Autodesk Inventor part; units mm, degrees
(part 3 of 6)
sketch "S06_305p5" plane through (0, 0, 0) normal (0, 0, 1) x (1, 0, 0)
  spline S0 degree 4 poles (213.0067, -18.9729) (212.9621, -18.9593) (212.7441, -18.8914) (212.3779, -18.779) (211.76, -18.589) (211.1099, -18.3887) (210.3111, -18.1449) (209.3704, -17.8569) (208.2858, -17.5275) (207.06, -17.1556) (205.6934, -16.744) (204.1871, -16.2917) (202.5432, -15.8012) (200.7622, -15.273) (198.8468, -14.7079) (196.7975, -14.1085) (194.6171, -13.4749) (192.3074, -12.8093) (189.8703, -12.1119) (187.3078, -11.3857) (184.6228, -10.6315) (181.8175, -9.8511) (178.8941, -9.0457) (175.8563, -8.2172) (172.7057, -7.3673) (169.4465, -6.4982) (166.0803, -5.6102) (162.6118, -4.7065) (159.0427, -3.7875) (155.3779, -2.8566) (151.6194, -1.9137) (147.7719, -0.9621) (143.8383, -0.0025) (139.823, 0.9626) (135.7291, 1.9321) (131.5615, 2.9039) (127.3228, 3.876) (123.0184, 4.8472) (118.6519, 5.8151) (114.2273, 6.7786) (109.7493, 7.7354) (105.2217, 8.684) (100.6494, 9.6229) (96.037, 10.5501) (91.388, 11.4635) (86.7084, 12.362) (82.0012, 13.2442) (77.2724, 14.1069) (72.5256, 14.9504) (67.7665, 15.7715) (62.9985, 16.5699) (58.2276, 17.3431) (53.4575, 18.0889) (48.6936, 18.8084) (43.9401, 19.497) (39.198, 20.1563) (34.4798, 20.7818) (29.764, 21.3777) (25.0643, 21.9267) (20.3983, 22.4316) (15.7673, 22.8898) (11.1792, 23.3003) (6.6388, 23.6643) (2.1513, 23.9785) (-2.2794, 24.2462) (-6.6474, 24.4635) (-10.9492, 24.6332) (-15.1794, 24.7536) (-19.3341, 24.8266) (-23.4084, 24.8507) (-27.3984, 24.828) (-31.2994, 24.7581) (-35.1072, 24.6427) (-38.8184, 24.4813) (-42.4284, 24.2766) (-45.9333, 24.0285) (-49.3303, 23.7389) (-52.6149, 23.4083) (-55.7842, 23.0395) (-58.8346, 22.6326) (-61.7632, 22.1892) (-64.5669, 21.7125) (-67.2427, 21.2022) (-69.788, 20.6607) (-72.2009, 20.0906) (-74.4779, 19.492) (-76.6177, 18.8678) (-78.6179, 18.2193) (-80.477, 17.548) (-82.1928, 16.8552) (-83.7647, 16.1431) (-85.1908, 15.4128) (-86.47, 14.6646) (-87.6028, 13.9015) (-88.5865, 13.1217) (-89.4223, 12.3271) (-90.1087, 11.5175) (-90.6444, 10.6919) (-91.026, 9.8504) (-91.2528, 8.9963) (-91.3206, 8.1309) (-91.2339, 7.2672) (-90.9897, 6.4183) (-90.5915, 5.5855) (-90.0424, 4.771) (-89.3451, 3.9743) (-88.5017, 3.1953) (-87.5133, 2.4322) (-86.3813, 1.6851) (-85.1065, 0.9538) (-83.6901, 0.2383) (-82.1338, -0.4608) (-80.4387, -1.1438) (-78.6069, -1.8099) (-76.64, -2.4594) (-74.5405, -3.091) (-72.3099, -3.7061) (-69.951, -4.3022) (-67.4659, -4.8811) (-64.8574, -5.442) (-62.1277, -5.9843) (-59.28, -6.5077) (-56.3167, -7.0143) (-53.2411, -7.5009) (-50.0561, -7.9709) (-46.7643, -8.422) (-43.3697, -8.8561) (-39.875, -9.2733) (-36.2838, -9.6725) (-32.5993, -10.0572) (-28.825, -10.4242) (-24.9649, -10.7779) (-21.0222, -11.1159) (-17.0003, -11.4409) (-12.9041, -11.7535) (-8.7359, -12.0531) (-4.5012, -12.3424) (-0.2027, -12.6213) (4.1549, -12.8906) (8.5679, -13.1521) (13.0318, -13.4068) (17.5428, -13.6542) (22.0992, -13.8979) (26.6939, -14.135) (31.334, -14.3737) (36.0271, -14.6) (40.7407, -14.8159) (45.4804, -15.0198) (50.2352, -15.2139) (55.002, -15.3986) (59.7756, -15.5745) (64.5509, -15.7416) (69.3235, -15.9018) (74.0888, -16.0537) (78.842, -16.2004) (83.5783, -16.3396) (88.2931, -16.4744) (92.9816, -16.6035) (97.6397, -16.727) (102.2619, -16.8472) (106.8441, -16.9625) (111.3818, -17.0733) (115.8706, -17.1813) (120.3053, -17.2848) (124.6826, -17.3854) (128.9972, -17.4825) (133.245, -17.576) (137.4219, -17.6663) (141.5241, -17.7536) (145.5464, -17.838) (149.4858, -17.9187) (153.338, -17.9962) (157.0988, -18.0714) (160.7646, -18.1421) (164.332, -18.2107) (167.7969, -18.2752) (171.156, -18.3377) (174.406, -18.3956) (177.5435, -18.4513) (180.565, -18.5032) (183.468, -18.5523) (186.2488, -18.5977) (188.9052, -18.641) (191.434, -18.6801) (193.8328, -18.7171) (196.0991, -18.7511) (198.2305, -18.7816) (200.2247, -18.81) (202.08, -18.836) (203.7939, -18.8588) (205.3647, -18.8797) (206.7912, -18.8976) (208.0711, -18.9142) (209.2039, -18.9279) (210.1875, -18.9398) (211.0222, -18.9501) (211.7026, -18.9575) (212.349, -18.9658) (212.7318, -18.9695) (212.96, -18.9722) (213.0067, -18.9729) knots 0 0 0 0 0 0.003306 0.005253 0.00752 0.010062 0.01285 0.015861 0.019079 0.022488 0.026078 0.029837 0.033757 0.037828 0.042045 0.046398 0.050884 0.055494 0.060224 0.065069 0.070023 0.075082 0.080241 0.085495 0.090841 0.096274 0.101791 0.107386 0.113057 0.118799 0.124609 0.130484 0.136419 0.142412 0.148458 0.154554 0.160697 0.166884 0.17311 0.179374 0.185671 0.191998 0.198352 0.20473 0.211128 0.217543 0.223972 0.230412 0.23686 0.243312 0.249765 0.256217 0.262663 0.2691 0.275526 0.281941 0.288345 0.294734 0.301105 0.307451 0.313767 0.320049 0.326294 0.332498 0.338659 0.344773 0.350837 0.356848 0.362801 0.368695 0.374525 0.380288 0.38598 0.391599 0.39714 0.4026 0.407976 0.413263 0.418458 0.423557 0.428556 0.433452 0.438241 0.442917 0.447478 0.451919 0.456236 0.460425 0.464482 0.468403 0.472185 0.475825 0.479322 0.482675 0.485889 0.48897 0.49193 0.494788 0.497572 0.50031 0.503032 0.505769 0.508552 0.511409 0.514365 0.517441 0.520647 0.523991 0.527474 0.531098 0.534861 0.538758 0.542789 0.546947 0.551231 0.555634 0.560154 0.564786 0.569527 0.574371 0.579315 0.584356 0.58949 0.594712 0.60002 0.605409 0.610877 0.61642 0.622034 0.627716 0.633463 0.639271 0.645138 0.651061 0.657035 0.663059 0.669128 0.675241 0.681393 0.687582 0.693804 0.700057 0.706341 0.712655 0.718998 0.725365 0.731751 0.738149 0.744556 0.750969 0.757385 0.7638 0.770211 0.776616 0.783011 0.789393 0.795759 0.802106 0.808429 0.814727 0.820996 0.827232 0.833433 0.839595 0.845714 0.851788 0.857813 0.863785 0.869702 0.875558 0.881352 0.887078 0.892735 0.898316 0.90382 0.909242 0.914577 0.919822 0.924972 0.930023 0.93497 0.939808 0.944533 0.949139 0.95362 0.95797 0.962183 0.966252 0.970169 0.973927 0.977515 0.980924 0.984141 0.987151 0.989939 0.99248 0.994747 0.996694 1 1 1 1 1
  circle A0 centre (0, 0) radius 5.15
  line L0 (-70.9, 8.1) -> (-60.7, 8.1)
  line L1 (-60.7, 8.1) -> (-60.7, 3.9)
  line L2 (-60.7, 3.9) -> (-70.9, 3.9)
  line L3 (-70.9, 3.9) -> (-70.9, 8.1)
  line L4 (-70.9, 8.1) -> (-60.7, 3.9) construction
  line L5 (-60.7, 8.1) -> (-70.9, 3.9) construction
  line L6 (-35.65, 7.1) -> (-25.45, 7.1)
  line L7 (-25.45, 7.1) -> (-25.45, 2.9)
  line L8 (-25.45, 2.9) -> (-35.65, 2.9)
  line L9 (-35.65, 2.9) -> (-35.65, 7.1)
  line L10 (-35.65, 7.1) -> (-25.45, 2.9) construction
  line L11 (-25.45, 7.1) -> (-35.65, 2.9) construction
  line L12 (120.1, -1.9) -> (109.9, -1.9)
  line L13 (109.9, -1.9) -> (109.9, -6.1)
  line L14 (109.9, -6.1) -> (120.1, -6.1)
  line L15 (120.1, -6.1) -> (120.1, -1.9)
  line L16 (120.1, -1.9) -> (109.9, -6.1) construction
  line L17 (109.9, -1.9) -> (120.1, -6.1) construction
  line L18 (59.1, -4.6) -> (48.9, -4.6)
  line L19 (48.9, -4.6) -> (48.9, -0.4)
  line L20 (48.9, -0.4) -> (59.1, -0.4)
  line L21 (59.1, -0.4) -> (59.1, -4.6)
  line L22 (59.1, -4.6) -> (48.9, -0.4) construction
  line L23 (48.9, -4.6) -> (59.1, -0.4) construction
  point P0 (212.7151, -18.8828)
  point P1 (212.3506, -18.7706)
  point P2 (211.841, -18.6139)
  point P3 (211.1866, -18.4126)
  point P4 (210.3879, -18.1682)
  point P5 (209.4456, -17.8803)
  point P6 (208.3604, -17.5502)
  point P7 (207.1336, -17.1784)
  point P8 (205.7662, -16.7662)
  point P9 (204.2591, -16.3139)
  point P10 (202.6141, -15.8229)
  point P11 (200.8323, -15.2943)
  point P12 (198.9157, -14.7292)
  point P13 (196.8654, -14.1291)
  point P14 (194.6838, -13.4953)
  point P15 (192.3729, -12.8291)
  point P16 (189.9344, -12.1316)
  point P17 (187.3706, -11.4048)
  point P18 (184.6842, -10.6503)
  point P19 (181.8775, -9.8693)
  point P20 (178.9527, -9.0635)
  point P21 (175.9131, -8.2345)
  point P22 (172.761, -7.3842)
  point P23 (169.5, -6.5144)
  point P24 (166.1323, -5.6262)
  point P25 (162.6618, -4.7217)
  point P26 (159.091, -3.8025)
  point P27 (155.4242, -2.8708)
  point P28 (151.6639, -1.9276)
  point P29 (147.8143, -0.9753)
  point P30 (143.8788, -0.0153)
  point P31 (139.8614, 0.9504)
  point P32 (135.7655, 1.9204)
  point P33 (131.5956, 2.8927)
  point P34 (127.3548, 3.8654)
  point P35 (123.0481, 4.837)
  point P36 (118.6794, 5.8055)
  point P37 (114.2526, 6.7693)
  point P38 (109.7722, 7.7266)
  point P39 (105.2423, 8.6757)
  point P40 (100.6677, 9.615)
  point P41 (96.0527, 10.5426)
  point P42 (91.4016, 11.4565)
  point P43 (86.7194, 12.3554)
  point P44 (82.0099, 13.2377)
  point P45 (77.2786, 14.1011)
  point P46 (72.5295, 14.9446)
  point P47 (67.7677, 15.7663)
  point P48 (62.9974, 16.5647)
  point P49 (58.2239, 17.338)
  point P50 (53.4515, 18.0845)
  point P51 (48.6851, 18.8035)
  point P52 (43.9294, 19.4928)
  point P53 (39.1892, 20.1511)
  point P54 (34.4692, 20.777)
  point P55 (29.7515, 21.3699)
  point P56 (25.0468, 21.9203)
  point P57 (20.3755, 22.425)
  point P58 (15.742, 22.8831)
  point P59 (11.1516, 23.2938)
  point P60 (6.6091, 23.657)
  point P61 (2.1192, 23.9717)
  point P62 (-2.3135, 24.2383)
  point P63 (-6.6837, 24.4558)
  point P64 (-10.9875, 24.6247)
  point P65 (-15.2198, 24.745)
  point P66 (-19.3763, 24.8171)
  point P67 (-23.4525, 24.841)
  point P68 (-27.4443, 24.8174)
  point P69 (-31.347, 24.747)
  point P70 (-35.1566, 24.6306)
  point P71 (-38.8693, 24.4687)
  point P72 (-42.4807, 24.2628)
  point P73 (-45.9871, 24.0139)
  point P74 (-49.3853, 23.7231)
  point P75 (-52.6712, 23.3916)
  point P76 (-55.8415, 23.0213)
  point P77 (-58.8928, 22.6131)
  point P78 (-61.8222, 22.1686)
  point P79 (-64.6265, 21.6899)
  point P80 (-67.3027, 21.1781)
  point P81 (-69.8483, 20.635)
  point P82 (-72.2609, 20.0626)
  point P83 (-74.5378, 19.4621)
  point P84 (-76.6767, 18.8356)
  point P85 (-78.6759, 18.1846)
  point P86 (-80.5332, 17.5106)
  point P87 (-82.2468, 16.8151)
  point P88 (-83.8155, 16.1001)
  point P89 (-85.2374, 15.3667)
  point P90 (-86.5115, 14.6162)
  point P91 (-87.6369, 13.8503)
  point P92 (-88.6122, 13.0695)
  point P93 (-89.4371, 12.2753)
  point P94 (-90.111, 11.4689)
  point P95 (-90.6333, 10.6504)
  point P96 (-91.0034, 9.821)
  point P97 (-91.2221, 8.981)
  point P98 (-91.2886, 8.1312)
  point P99 (-91.2037, 7.283)
  point P100 (-90.9677, 6.448)
  point P101 (-90.5814, 5.6265)
  point P102 (-90.0455, 4.8188)
  point P103 (-89.3605, 4.025)
  point P104 (-88.5275, 3.246)
  point P105 (-87.5476, 2.4815)
  point P106 (-86.4222, 1.732)
  point P107 (-85.1524, 0.9978)
  point P108 (-83.7399, 0.2794)
  point P109 (-82.1864, -0.4227)
  point P110 (-80.4934, -1.1084)
  point P111 (-78.663, -1.7772)
  point P112 (-76.6971, -2.4289)
  point P113 (-74.5981, -3.0631)
  point P114 (-72.3677, -3.6798)
  point P115 (-70.0087, -4.2782)
  point P116 (-67.5233, -4.8587)
  point P117 (-64.9143, -5.4212)
  point P118 (-62.1839, -5.9649)
  point P119 (-59.3353, -6.4901)
  point P120 (-56.3711, -6.9973)
  point P121 (-53.2944, -7.4858)
  point P122 (-50.1082, -7.9564)
  point P123 (-46.8152, -8.4089)
  point P124 (-43.4191, -8.8439)
  point P125 (-39.9231, -9.2617)
  point P126 (-36.3304, -9.6624)
  point P127 (-32.6443, -10.0471)
  point P128 (-28.8684, -10.4156)
  point P129 (-25.0065, -10.7694)
  point P130 (-21.0621, -11.1085)
  point P131 (-17.0385, -11.4341)
  point P132 (-12.9402, -11.747)
  point P133 (-8.7703, -12.0476)
  point P134 (-4.5334, -12.3372)
  point P135 (-0.2331, -12.6166)
  point P136 (4.1267, -12.8865)
  point P137 (8.5417, -13.1485)
  point P138 (13.0077, -13.4034)
  point P139 (17.5206, -13.6517)
  point P140 (22.0763, -13.8949)
  point P141 (26.6704, -14.1336)
  point P142 (31.3138, -14.3696)
  point P143 (36.0095, -14.5968)
  point P144 (40.7302, -14.8127)
  point P145 (45.4721, -15.0173)
  point P146 (50.2296, -15.2116)
  point P147 (54.9987, -15.3966)
  point P148 (59.7748, -15.5726)
  point P149 (64.5525, -15.7402)
  point P150 (69.3275, -15.9003)
  point P151 (74.0952, -16.0529)
  point P152 (78.8509, -16.1992)
  point P153 (83.5897, -16.3391)
  point P154 (88.3068, -16.4737)
  point P155 (92.9978, -16.603)
  point P156 (97.6582, -16.727)
  point P157 (102.2829, -16.8469)
  point P158 (106.8674, -16.9624)
  point P159 (111.4075, -17.0736)
  point P160 (115.8986, -17.1813)
  point P161 (120.3357, -17.2852)
  point P162 (124.7151, -17.3857)
  point P163 (129.032, -17.4828)
  point P164 (133.282, -17.5765)
  point P165 (137.4612, -17.6668)
  point P166 (141.5654, -17.7542)
  point P167 (145.5899, -17.8385)
  point P168 (149.5313, -17.9193)
  point P169 (153.3856, -17.997)
  point P170 (157.1484, -18.0718)
  point P171 (160.8161, -18.143)
  point P172 (164.3853, -18.2113)
  point P173 (167.8521, -18.2762)
  point P174 (171.213, -18.3382)
  point P175 (174.4648, -18.3966)
  point P176 (177.6039, -18.452)
  point P177 (180.6271, -18.5041)
  point P178 (183.5316, -18.553)
  point P179 (186.314, -18.5987)
  point P180 (188.9718, -18.6416)
  point P181 (191.502, -18.6811)
  point P182 (193.9021, -18.7179)
  point P183 (196.1696, -18.7518)
  point P184 (198.3022, -18.7826)
  point P185 (200.2976, -18.811)
  point P186 (202.1539, -18.8368)
  point P187 (203.8689, -18.8598)
  point P188 (205.4407, -18.8805)
  point P189 (206.8681, -18.8987)
  point P190 (208.149, -18.915)
  point P191 (209.2826, -18.9288)
  point P192 (210.2676, -18.9408)
  point P193 (211.1025, -18.9508)
  point P194 (211.7873, -18.9587)
  point P195 (212.3204, -18.9651)
  point P196 (212.7015, -18.9693)
  point P197 (212.9304, -18.9719)
  point P198 (-65.8, 6)
  point P199 (-30.55, 5)
  dimension "d10" = 10.3
  dimension "d11" = 91.65
  dimension "d69" = 10.2
  dimension "d70" = 4.2
  dimension "d72" = 10.2
  dimension "d73" = 4.2
  dimension "d142" = 65.8
  dimension "d143" = 6
  dimension "d144" = 0
  dimension "d145" = 30.55
  dimension "d146" = 5
  dimension "d227" = 10.2
  dimension "d228" = 4.2
  dimension "d229" = 115
  dimension "d230" = 4
  dimension "d231" = 10.2
  dimension "d232" = 4.2
  dimension "d233" = 54
  dimension "d234" = 2.5
  constraints: 48 end point, 8 midpoint, 8 parallel, 4 horizontal, 4 perpendicular, 1 centre point, 201 other
  measures "d10" diameter of A0
  measures "d11" distance of A0.centre point (-91.289, 8.131)
  measures "d69" distance of L1.end L2.end
  measures "d70" distance of L0.end L1.end
  measures "d72" distance of L7.end L8.end
  measures "d73" distance of L6.end L7.end
  measures "d142" horizontal distance of point (0, 0) point (-65.8, 6)
  measures "d143" vertical distance of A0.centre point (-65.8, 6)
  measures "d144" distance of point (0, 0) A0.centre
  measures "d145" horizontal distance of point (0, 0) point (-30.55, 5)
  measures "d146" vertical distance of point (0, 0) point (-30.55, 5)
  measures "d227" distance of L14.end L13.end
  measures "d228" distance of L13.end L12.end
  measures "d229" horizontal distance of point (0, 0) point (115, -4)
  measures "d230" vertical distance of point (115, -4) point (0, 0)
  measures "d231" distance of L19.end L20.end
  measures "d232" distance of L18.end L19.end
  measures "d233" horizontal distance of point (54, -2.5) point (0, 0)
  measures "d234" vertical distance of point (0, 0) point (54, -2.5)
sketch "S07_285p6" plane through (0, 0, 0) normal (0, 0, 1) x (1, 0, 0)
  spline S0 degree 4 poles (198.678, -22.2502) (198.6365, -22.2366) (198.4342, -22.1685) (198.0944, -22.0557) (197.5209, -21.865) (196.9176, -21.664) (196.1762, -21.4192) (195.3031, -21.13) (194.2964, -20.7992) (193.1586, -20.4256) (191.8901, -20.0119) (190.4919, -19.5573) (188.9658, -19.0639) (187.3125, -18.5325) (185.5343, -17.9638) (183.6317, -17.3601) (181.6073, -16.7216) (179.4627, -16.0506) (177.1997, -15.3471) (174.8202, -14.614) (172.3267, -13.8522) (169.7214, -13.0633) (167.0062, -12.2486) (164.1846, -11.4098) (161.258, -10.5486) (158.2303, -9.6672) (155.103, -8.7659) (151.8805, -7.8477) (148.5642, -6.9131) (145.1587, -5.9654) (141.666, -5.0044) (138.0902, -4.0334) (134.4342, -3.0531) (130.7019, -2.0659) (126.8961, -1.073) (123.0216, -0.0763) (119.0807, 0.9221) (115.0783, 1.9211) (111.0178, 2.9184) (106.9029, 3.9127) (102.738, 4.9019) (98.5265, 5.8845) (94.2731, 6.859) (89.9818, 7.8235) (85.6562, 8.7757) (81.3016, 9.7147) (76.9209, 10.6391) (72.5196, 11.5457) (68.101, 12.4347) (63.6704, 13.3031) (59.2311, 14.1504) (54.7886, 14.9742) (50.3461, 15.7725) (45.9089, 16.5459) (41.4808, 17.2904) (37.0628, 18.0071) (32.6663, 18.6918) (28.2715, 19.3488) (23.8906, 19.9616) (19.5404, 20.5324) (15.2219, 21.0589) (10.9425, 21.5399) (6.7067, 21.9763) (2.5193, 22.3652) (-1.6161, 22.7093) (-5.6939, 23.0051) (-9.7109, 23.2549) (-13.662, 23.4572) (-17.5435, 23.6135) (-21.3509, 23.7225) (-25.0805, 23.7859) (-28.7279, 23.8033) (-32.2893, 23.7762) (-35.7612, 23.7041) (-39.1395, 23.5893) (-42.4206, 23.4317) (-45.6016, 23.2331) (-48.6785, 22.9938) (-51.6484, 22.7163) (-54.508, 22.4008) (-57.2545, 22.0485) (-59.885, 21.6624) (-62.3967, 21.2422) (-64.7871, 20.7901) (-67.0543, 20.3084) (-69.1952, 19.7973) (-71.2083, 19.2592) (-73.0915, 18.6956) (-74.8433, 18.1076) (-76.4615, 17.4965) (-77.9458, 16.8643) (-79.2942, 16.212) (-80.5056, 15.5398) (-81.5805, 14.8506) (-82.5165, 14.1427) (-83.3144, 13.4177) (-83.9732, 12.6757) (-84.4913, 11.9154) (-84.8658, 11.137) (-85.0959, 10.3436) (-85.1776, 9.5362) (-85.1149, 8.7271) (-84.9046, 7.9286) (-84.5502, 7.1417) (-84.0543, 6.3688) (-83.4195, 5.6094) (-82.6477, 4.8635) (-81.7401, 4.1293) (-80.698, 3.407) (-79.522, 2.6965) (-78.2134, 1.9977) (-76.7737, 1.3113) (-75.2039, 0.637) (-73.506, -0.0244) (-71.6815, -0.6731) (-69.7326, -1.308) (-67.6609, -1.9301) (-65.4689, -2.5373) (-63.1585, -3.1311) (-60.7325, -3.7106) (-58.1927, -4.2754) (-55.5423, -4.8249) (-52.7835, -5.3613) (-49.9193, -5.8813) (-46.9525, -6.3881) (-43.8855, -6.8795) (-40.722, -7.3572) (-37.4646, -7.8213) (-34.1167, -8.2706) (-30.6813, -8.7082) (-27.1615, -9.1313) (-23.5613, -9.5438) (-19.8835, -9.9433) (-16.1315, -10.3323) (-12.3098, -10.7113) (-8.4204, -11.0798) (-4.4687, -11.44) (-0.4572, -11.7918) (3.6099, -12.1359) (7.7288, -12.4739) (11.8955, -12.8067) (16.1063, -13.1336) (20.3596, -13.4579) (24.6488, -13.7771) (28.9806, -14.0985) (33.362, -14.4096) (37.7628, -14.7113) (42.1883, -15.0025) (46.6281, -15.2847) (51.0794, -15.5584) (55.5372, -15.8241) (59.9967, -16.0815) (64.4539, -16.3324) (68.9044, -16.5755) (73.3437, -16.8134) (77.7674, -17.044) (82.1711, -17.2699) (86.5503, -17.4901) (90.9013, -17.7043) (95.2187, -17.9147) (99.4989, -18.1196) (103.7376, -18.3194) (107.9306, -18.5156) (112.0732, -18.7063) (116.1622, -18.8932) (120.1926, -19.0755) (124.1607, -19.253) (128.0626, -19.4259) (131.8948, -19.5946) (135.6523, -19.7587) (139.3324, -19.9177) (142.9311, -20.0718) (146.4444, -20.2218) (149.869, -20.3657) (153.2017, -20.5055) (156.4387, -20.6393) (159.5769, -20.7689) (162.6132, -20.8919) (165.5444, -21.0105) (168.3673, -21.1232) (171.0794, -21.2306) (173.6774, -21.332) (176.1593, -21.4289) (178.5219, -21.519) (180.7631, -21.6044) (182.8805, -21.6844) (184.8719, -21.758) (186.7351, -21.8269) (188.4685, -21.8905) (190.0699, -21.9481) (191.5376, -22.0011) (192.8705, -22.0481) (194.0663, -22.0907) (195.1248, -22.1275) (196.0438, -22.1595) (196.8237, -22.1868) (197.4594, -22.2081) (198.0634, -22.2296) (198.4212, -22.2412) (198.6343, -22.2486) (198.678, -22.2502) knots 0 0 0 0 0 0.003306 0.005253 0.00752 0.010062 0.01285 0.015861 0.019079 0.022488 0.026078 0.029837 0.033757 0.037828 0.042045 0.046398 0.050884 0.055494 0.060224 0.065069 0.070023 0.075082 0.080241 0.085495 0.090841 0.096274 0.101791 0.107386 0.113057 0.118799 0.124609 0.130484 0.136419 0.142412 0.148458 0.154554 0.160697 0.166884 0.17311 0.179374 0.185671 0.191998 0.198352 0.20473 0.211128 0.217543 0.223972 0.230412 0.23686 0.243312 0.249765 0.256217 0.262663 0.2691 0.275526 0.281941 0.288345 0.294734 0.301105 0.307451 0.313767 0.320049 0.326294 0.332498 0.338659 0.344773 0.350837 0.356848 0.362801 0.368695 0.374525 0.380288 0.38598 0.391599 0.39714 0.4026 0.407976 0.413263 0.418458 0.423557 0.428556 0.433452 0.438241 0.442917 0.447478 0.451919 0.456236 0.460425 0.464482 0.468403 0.472185 0.475825 0.479322 0.482675 0.485889 0.48897 0.49193 0.494788 0.497572 0.50031 0.503032 0.505769 0.508552 0.511409 0.514365 0.517441 0.520647 0.523991 0.527474 0.531098 0.534861 0.538758 0.542789 0.546947 0.551231 0.555634 0.560154 0.564786 0.569527 0.574371 0.579315 0.584356 0.58949 0.594712 0.60002 0.605409 0.610877 0.61642 0.622034 0.627716 0.633463 0.639271 0.645138 0.651061 0.657035 0.663059 0.669128 0.675241 0.681393 0.687582 0.693804 0.700057 0.706341 0.712655 0.718998 0.725365 0.731751 0.738149 0.744556 0.750969 0.757385 0.7638 0.770211 0.776616 0.783011 0.789393 0.795759 0.802106 0.808429 0.814727 0.820996 0.827232 0.833433 0.839595 0.845714 0.851788 0.857813 0.863785 0.869702 0.875558 0.881352 0.887078 0.892735 0.898316 0.90382 0.909242 0.914577 0.919822 0.924972 0.930023 0.93497 0.939808 0.944533 0.949139 0.95362 0.95797 0.962183 0.966252 0.970169 0.973927 0.977515 0.980924 0.984141 0.987151 0.989939 0.99248 0.994747 0.996694 1 1 1 1 1
  circle A0 centre (0, 0) radius 5.15
  line L0 (-25.45, 2.9) -> (-35.65, 2.9)
  line L1 (-35.65, 2.9) -> (-35.65, 7.1)
  line L2 (-35.65, 7.1) -> (-25.45, 7.1)
  line L3 (-25.45, 7.1) -> (-25.45, 2.9)
  line L4 (-25.45, 2.9) -> (-35.65, 7.1) construction
  line L5 (-35.65, 2.9) -> (-25.45, 7.1) construction
  line L6 (-62.22, 12.1) -> (-52.02, 12.1)
  line L7 (-52.02, 12.1) -> (-52.02, 7.9)
  line L8 (-52.02, 7.9) -> (-62.22, 7.9)
  line L9 (-62.22, 7.9) -> (-62.22, 12.1)
  line L10 (-62.22, 12.1) -> (-52.02, 7.9) construction
  line L11 (-52.02, 12.1) -> (-62.22, 7.9) construction
  line L12 (48.9, -0.4) -> (59.1, -0.4)
  line L13 (59.1, -0.4) -> (59.1, -4.6)
  line L14 (59.1, -4.6) -> (48.9, -4.6)
  line L15 (48.9, -4.6) -> (48.9, -0.4)
  line L16 (48.9, -0.4) -> (59.1, -4.6) construction
  line L17 (59.1, -0.4) -> (48.9, -4.6) construction
  line L18 (105.1, -12.1) -> (94.9, -12.1)
  line L19 (94.9, -12.1) -> (94.9, -7.9)
  line L20 (94.9, -7.9) -> (105.1, -7.9)
  line L21 (105.1, -7.9) -> (105.1, -12.1)
  line L22 (105.1, -12.1) -> (94.9, -7.9) construction
  line L23 (94.9, -12.1) -> (105.1, -7.9) construction
  point P0 (198.4073, -22.1598)
  point P1 (198.069, -22.0472)
  point P2 (197.5961, -21.8899)
  point P3 (196.9887, -21.688)
  point P4 (196.2475, -21.4426)
  point P5 (195.3729, -21.1535)
  point P6 (194.3656, -20.822)
  point P7 (193.2269, -20.4485)
  point P8 (191.9576, -20.0342)
  point P9 (190.5587, -19.5795)
  point P10 (189.0316, -19.0858)
  point P11 (187.3775, -18.5539)
  point P12 (185.5982, -17.9851)
  point P13 (183.6947, -17.3808)
  point P14 (181.6692, -16.7421)
  point P15 (179.5235, -16.0705)
  point P16 (177.2592, -15.3668)
  point P17 (174.8785, -14.6332)
  point P18 (172.3837, -13.871)
  point P19 (169.777, -13.0816)
  point P20 (167.0606, -12.2664)
  point P21 (164.2373, -11.4272)
  point P22 (161.3093, -10.5656)
  point P23 (158.2799, -9.6835)
  point P24 (155.1513, -8.7819)
  point P25 (151.9268, -7.863)
  point P26 (148.6091, -6.9281)
  point P27 (145.2017, -5.9795)
  point P28 (141.7073, -5.0183)
  point P29 (138.1295, -4.0466)
  point P30 (134.4717, -3.0659)
  point P31 (130.7374, -2.0781)
  point P32 (126.9299, -1.0847)
  point P33 (123.0532, -0.0875)
  point P34 (119.1104, 0.9115)
  point P35 (115.1058, 1.9109)
  point P36 (111.0433, 2.9088)
  point P37 (106.9264, 3.9035)
  point P38 (102.7592, 4.8932)
  point P39 (98.5456, 5.8764)
  point P40 (94.29, 6.8513)
  point P41 (89.9964, 7.8161)
  point P42 (85.6688, 8.7689)
  point P43 (81.3118, 9.7083)
  point P44 (76.9289, 10.6328)
  point P45 (72.5252, 11.5402)
  point P46 (68.1045, 12.4292)
  point P47 (63.6714, 13.2981)
  point P48 (59.23, 14.1456)
  point P49 (54.785, 14.9696)
  point P50 (50.3404, 15.7685)
  point P51 (45.9009, 16.5416)
  point P52 (41.4707, 17.2866)
  point P53 (37.0544, 18.0025)
  point P54 (32.6563, 18.6876)
  point P55 (28.2596, 19.3418)
  point P56 (23.8741, 19.9559)
  point P57 (19.5189, 20.5267)
  point P58 (15.1981, 21.0531)
  point P59 (10.9165, 21.5343)
  point P60 (6.6787, 21.9701)
  point P61 (2.4891, 22.3595)
  point P62 (-1.6482, 22.7027)
  point P63 (-5.7281, 22.9986)
  point P64 (-9.7468, 23.2478)
  point P65 (-13.6999, 23.45)
  point P66 (-17.5831, 23.6055)
  point P67 (-21.3923, 23.7143)
  point P68 (-25.1236, 23.777)
  point P69 (-28.7727, 23.7939)
  point P70 (-32.3357, 23.7659)
  point P71 (-35.8091, 23.6933)
  point P72 (-39.1888, 23.5775)
  point P73 (-42.4712, 23.4192)
  point P74 (-45.6534, 23.2195)
  point P75 (-48.7314, 22.9794)
  point P76 (-51.7023, 22.7005)
  point P77 (-54.5628, 22.3838)
  point P78 (-57.3101, 22.0304)
  point P79 (-59.9412, 21.6426)
  point P80 (-62.4533, 21.2209)
  point P81 (-64.844, 20.7673)
  point P82 (-67.111, 20.2835)
  point P83 (-69.2517, 19.7706)
  point P84 (-71.2641, 19.2304)
  point P85 (-73.1464, 18.6644)
  point P86 (-74.8966, 18.0738)
  point P87 (-76.5129, 17.4602)
  point P88 (-77.9942, 16.8251)
  point P89 (-79.3387, 16.1699)
  point P90 (-80.5454, 15.4955)
  point P91 (-81.6135, 14.8035)
  point P92 (-82.5416, 14.0944)
  point P93 (-83.3294, 13.3696)
  point P94 (-83.9764, 12.6302)
  point P95 (-84.4818, 11.8764)
  point P96 (-84.8454, 11.109)
  point P97 (-85.0675, 10.3286)
  point P98 (-85.1477, 9.5358)
  point P99 (-85.0864, 8.7412)
  point P100 (-84.8835, 7.9558)
  point P101 (-84.5399, 7.1799)
  point P102 (-84.0561, 6.4135)
  point P103 (-83.4327, 5.6572)
  point P104 (-82.6707, 4.9114)
  point P105 (-81.7711, 4.1761)
  point P106 (-80.7352, 3.4517)
  point P107 (-79.564, 2.7386)
  point P108 (-78.2591, 2.0372)
  point P109 (-76.8221, 1.3481)
  point P110 (-75.2543, 0.6713)
  point P111 (-73.5578, 0.0074)
  point P112 (-71.7342, -0.6434)
  point P113 (-69.7858, -1.2806)
  point P114 (-67.7144, -1.9043)
  point P115 (-65.5223, -2.5136)
  point P116 (-63.2117, -3.1089)
  point P117 (-60.7852, -3.6899)
  point P118 (-58.2448, -4.2561)
  point P119 (-55.5937, -4.8073)
  point P120 (-52.834, -5.3443)
  point P121 (-49.9688, -5.866)
  point P122 (-47.0009, -6.3734)
  point P123 (-43.9328, -6.8662)
  point P124 (-40.768, -7.3447)
  point P125 (-37.5093, -7.8094)
  point P126 (-34.16, -8.2601)
  point P127 (-30.7231, -8.6979)
  point P128 (-27.2019, -9.1224)
  point P129 (-23.6, -9.535)
  point P130 (-19.9206, -9.9355)
  point P131 (-16.167, -10.3251)
  point P132 (-12.3433, -10.7045)
  point P133 (-8.4524, -11.0739)
  point P134 (-4.4987, -11.4345)
  point P135 (-0.4854, -11.7868)
  point P136 (3.5835, -12.1315)
  point P137 (7.7044, -12.47)
  point P138 (11.873, -12.803)
  point P139 (16.0856, -13.1307)
  point P140 (20.3382, -13.4547)
  point P141 (24.6269, -13.7752)
  point P142 (28.9617, -14.0943)
  point P143 (33.3456, -14.4062)
  point P144 (37.7531, -14.7081)
  point P145 (42.1806, -14.9999)
  point P146 (46.623, -15.2824)
  point P147 (51.0764, -15.5564)
  point P148 (55.5364, -15.8223)
  point P149 (59.9982, -16.0803)
  point P150 (64.4577, -16.3311)
  point P151 (68.9104, -16.5749)
  point P152 (73.3521, -16.8125)
  point P153 (77.7781, -17.0438)
  point P154 (82.184, -17.2696)
  point P155 (86.5655, -17.4899)
  point P156 (90.9186, -17.7047)
  point P157 (95.2383, -17.9149)
  point P158 (99.5207, -18.12)
  point P159 (103.7616, -18.3202)
  point P160 (107.9567, -18.5161)
  point P161 (112.1016, -18.7073)
  point P162 (116.1925, -18.8942)
  point P163 (120.2251, -19.0765)
  point P164 (124.1953, -19.2542)
  point P165 (128.0993, -19.4273)
  point P166 (131.9334, -19.596)
  point P167 (135.693, -19.7601)
  point P168 (139.3749, -19.9193)
  point P169 (142.9755, -20.0736)
  point P170 (146.4907, -20.2233)
  point P171 (149.9172, -20.3676)
  point P172 (153.2516, -20.5071)
  point P173 (156.4903, -20.6414)
  point P174 (159.6302, -20.7706)
  point P175 (162.6681, -20.8941)
  point P176 (165.6009, -21.0125)
  point P177 (168.4253, -21.1253)
  point P178 (171.1388, -21.2326)
  point P179 (173.7383, -21.3344)
  point P180 (176.2215, -21.4308)
  point P181 (178.5854, -21.5214)
  point P182 (180.8278, -21.6067)
  point P183 (182.9464, -21.6865)
  point P184 (184.9389, -21.7605)
  point P185 (186.8032, -21.8293)
  point P186 (188.5377, -21.8928)
  point P187 (190.14, -21.9507)
  point P188 (191.6086, -22.0034)
  point P189 (192.9423, -22.0507)
  point P190 (194.1391, -22.0931)
  point P191 (195.1983, -22.1301)
  point P192 (196.1186, -22.1622)
  point P193 (196.8987, -22.1892)
  point P194 (197.5386, -22.2111)
  point P195 (198.0367, -22.2284)
  point P196 (198.3928, -22.2404)
  point P197 (198.6067, -22.2477)
  point P198 (-30.55, 5)
  point P199 (-57.12, 10)
  dimension "d12" = 10.3
  dimension "d13" = 85.68
  dimension "d75" = 10.2
  dimension "d76" = 4.2
  dimension "d78" = 10.2
  dimension "d79" = 4.2
  dimension "d147" = 30.55
  dimension "d148" = 5
  dimension "d149" = 57.12
  dimension "d150" = 10
  dimension "d235" = 10.2
  dimension "d236" = 4.2
  dimension "d237" = 54
  dimension "d238" = 2.5
  dimension "d239" = 10.2
  dimension "d240" = 4.2
  dimension "d241" = 100
  dimension "d242" = 10
  constraints: 48 end point, 8 midpoint, 8 parallel, 4 horizontal, 4 perpendicular, 1 centre point, 201 other
  measures "d12" diameter of A0
  measures "d13" distance of A0.centre point (-85.148, 9.536)
  measures "d75" distance of L1.end L2.end
  measures "d76" distance of L0.end L1.end
  measures "d78" distance of L7.end L8.end
  measures "d79" distance of L6.end L7.end
  measures "d147" horizontal distance of point (0, 0) point (-30.55, 5)
  measures "d148" vertical distance of point (0, 0) point (-30.55, 5)
  measures "d149" horizontal distance of point (0, 0) point (-57.12, 10)
  measures "d150" vertical distance of point (0, 0) point (-57.12, 10)
  measures "d235" distance of L13.end L14.end
  measures "d236" distance of L12.end L13.end
  measures "d237" horizontal distance of point (0, 0) point (54, -2.5)
  measures "d238" vertical distance of point (0, 0) point (54, -2.5)
  measures "d239" distance of L19.end L20.end
  measures "d240" distance of L18.end L19.end
  measures "d241" horizontal distance of point (100, -10) point (0, 0)
  measures "d242" vertical distance of point (0, 0) point (100, -10)
sketch "S08_271p4" plane through (0, 0, 0) normal (0, 0, 1) x (1, 0, 0)
  spline S0 degree 4 poles (187.5255, -30.4397) (187.4869, -30.4248) (187.298, -30.3507) (186.9808, -30.2277) (186.4454, -30.0198) (185.8822, -29.8007) (185.19, -29.5336) (184.375, -29.2182) (183.435, -28.857) (182.3726, -28.449) (181.188, -27.9968) (179.8823, -27.4997) (178.457, -26.9599) (176.9127, -26.3779) (175.2517, -25.7547) (173.4742, -25.0924) (171.5828, -24.3915) (169.5788, -23.6539) (167.4639, -22.8801) (165.2399, -22.0727) (162.909, -21.2326) (160.4732, -20.3617) (157.9345, -19.461) (155.2958, -18.5325) (152.5584, -17.5778) (149.7261, -16.5992) (146.8003, -15.597) (143.7848, -14.5743) (140.6811, -13.5317) (137.4934, -12.4724) (134.2234, -11.3964) (130.8751, -10.3071) (127.4511, -9.2051) (123.955, -8.0931) (120.3895, -6.9721) (116.7589, -5.8443) (113.0653, -4.7118) (109.3133, -3.5759) (105.5063, -2.4388) (101.6474, -1.302) (97.7408, -0.1678) (93.7897, 0.9625) (89.7984, 2.0869) (85.7707, 3.2037) (81.7099, 4.3104) (77.6209, 5.4059) (73.5064, 6.4889) (69.3716, 7.5558) (65.2195, 8.6069) (61.0551, 9.639) (56.8814, 10.6514) (52.7036, 11.6418) (48.5246, 12.6079) (44.3494, 13.5501) (40.1815, 14.4645) (36.0219, 15.352) (31.8812, 16.2082) (27.7409, 17.0379) (23.6116, 17.825) (19.5095, 18.5709) (15.4354, 19.2732) (11.3964, 19.9305) (7.3966, 20.5435) (3.4404, 21.1091) (-0.4684, 21.6297) (-4.3249, 22.1017) (-8.1257, 22.5274) (-11.8663, 22.9047) (-15.543, 23.2352) (-19.1515, 23.5172) (-22.6884, 23.7524) (-26.1495, 23.9401) (-29.5309, 24.0814) (-32.8296, 24.1759) (-36.0414, 24.2254) (-39.1629, 24.2298) (-42.1914, 24.1906) (-45.1229, 24.1078) (-47.9548, 23.9838) (-50.6837, 23.8184) (-53.307, 23.6129) (-55.8218, 23.3699) (-58.2254, 23.0889) (-60.5154, 22.772) (-62.6898, 22.4212) (-64.7458, 22.0365) (-66.6817, 21.6203) (-68.4955, 21.1737) (-70.1858, 20.6978) (-71.7504, 20.1937) (-73.1888, 19.6633) (-74.4991, 19.1075) (-75.6805, 18.5264) (-76.733, 17.9227) (-77.6546, 17.2946) (-78.446, 16.644) (-79.106, 15.9706) (-79.6335, 15.2733) (-80.0254, 14.5521) (-80.281, 13.8098) (-80.3965, 13.0474) (-80.3749, 12.2765) (-80.2128, 11.5087) (-79.9133, 10.7452) (-79.4789, 9.9884) (-78.912, 9.2379) (-78.2145, 8.4937) (-77.3875, 7.7543) (-76.4323, 7.0199) (-75.3495, 6.2903) (-74.1403, 5.5657) (-72.806, 4.8467) (-71.3477, 4.133) (-69.7673, 3.4256) (-68.066, 2.7243) (-66.2461, 2.0303) (-64.3089, 1.3426) (-62.257, 0.6634) (-60.092, -0.0085) (-57.8166, -0.6724) (-55.4325, -1.3276) (-52.9428, -1.9735) (-50.3495, -2.612) (-47.6554, -3.2399) (-44.8633, -3.8601) (-41.9754, -4.4705) (-38.9953, -5.0723) (-35.9254, -5.6656) (-32.7689, -6.2491) (-29.5288, -6.8257) (-26.208, -7.3924) (-22.8103, -7.9527) (-19.3384, -8.5045) (-15.7955, -9.0497) (-12.186, -9.5888) (-8.5118, -10.121) (-4.778, -10.6483) (-0.9872, -11.1704) (2.8568, -11.6878) (6.7503, -12.2019) (10.6894, -12.7132) (14.6706, -13.221) (18.6923, -13.7284) (22.7483, -14.2326) (26.8446, -14.7409) (30.9885, -15.2417) (35.1513, -15.7345) (39.338, -16.2185) (43.5386, -16.6947) (47.7506, -17.1633) (51.9691, -17.6246) (56.1896, -18.0783) (60.4083, -18.5255) (64.6209, -18.965) (68.8232, -19.3991) (73.011, -19.8255) (77.1801, -20.2466) (81.3261, -20.661) (85.4457, -21.0684) (89.5336, -21.4706) (93.5864, -21.866) (97.6, -22.2545) (101.5705, -22.6374) (105.4934, -23.0128) (109.3655, -23.382) (113.1823, -23.7441) (116.9403, -24.0987) (120.6355, -24.446) (124.2648, -24.7858) (127.8234, -25.1179) (131.3088, -25.4415) (134.7172, -25.7566) (138.0447, -26.0639) (141.2884, -26.361) (144.4449, -26.6501) (147.511, -26.929) (150.4834, -27.1992) (153.3594, -27.4585) (156.1359, -27.7085) (158.8099, -27.9479) (161.379, -28.1771) (163.8401, -28.3952) (166.1911, -28.6036) (168.4293, -28.8) (170.5524, -28.9863) (172.5583, -29.1615) (174.445, -29.3248) (176.2101, -29.4776) (177.8524, -29.6193) (179.3696, -29.7491) (180.7601, -29.8682) (182.023, -29.9754) (183.156, -30.072) (184.1589, -30.1565) (185.0297, -30.2301) (185.7685, -30.2925) (186.371, -30.3426) (186.9432, -30.3913) (187.2822, -30.4191) (187.4842, -30.4361) (187.5255, -30.4397) knots 0 0 0 0 0 0.003306 0.005253 0.00752 0.010062 0.01285 0.015861 0.019079 0.022488 0.026078 0.029837 0.033757 0.037828 0.042045 0.046398 0.050884 0.055494 0.060224 0.065069 0.070023 0.075082 0.080241 0.085495 0.090841 0.096274 0.101791 0.107386 0.113057 0.118799 0.124609 0.130484 0.136419 0.142412 0.148458 0.154554 0.160697 0.166884 0.17311 0.179374 0.185671 0.191998 0.198352 0.20473 0.211128 0.217543 0.223972 0.230412 0.23686 0.243312 0.249765 0.256217 0.262663 0.2691 0.275526 0.281941 0.288345 0.294734 0.301105 0.307451 0.313767 0.320049 0.326294 0.332498 0.338659 0.344773 0.350837 0.356848 0.362801 0.368695 0.374525 0.380288 0.38598 0.391599 0.39714 0.4026 0.407976 0.413263 0.418458 0.423557 0.428556 0.433452 0.438241 0.442917 0.447478 0.451919 0.456236 0.460425 0.464482 0.468403 0.472185 0.475825 0.479322 0.482675 0.485889 0.48897 0.49193 0.494788 0.497572 0.50031 0.503032 0.505769 0.508552 0.511409 0.514365 0.517441 0.520647 0.523991 0.527474 0.531098 0.534861 0.538758 0.542789 0.546947 0.551231 0.555634 0.560154 0.564786 0.569527 0.574371 0.579315 0.584356 0.58949 0.594712 0.60002 0.605409 0.610877 0.61642 0.622034 0.627716 0.633463 0.639271 0.645138 0.651061 0.657035 0.663059 0.669128 0.675241 0.681393 0.687582 0.693804 0.700057 0.706341 0.712655 0.718998 0.725365 0.731751 0.738149 0.744556 0.750969 0.757385 0.7638 0.770211 0.776616 0.783011 0.789393 0.795759 0.802106 0.808429 0.814727 0.820996 0.827232 0.833433 0.839595 0.845714 0.851788 0.857813 0.863785 0.869702 0.875558 0.881352 0.887078 0.892735 0.898316 0.90382 0.909242 0.914577 0.919822 0.924972 0.930023 0.93497 0.939808 0.944533 0.949139 0.95362 0.95797 0.962183 0.966252 0.970169 0.973927 0.977515 0.980924 0.984141 0.987151 0.989939 0.99248 0.994747 0.996694 1 1 1 1 1
  circle A0 centre (0, 0) radius 5.15
  line L0 (-62.22, 7.9) -> (-52.02, 7.9)
  line L1 (-52.02, 7.9) -> (-52.02, 12.1)
  line L2 (-52.02, 12.1) -> (-62.22, 12.1)
  line L3 (-62.22, 12.1) -> (-62.22, 7.9)
  line L4 (-62.22, 7.9) -> (-52.02, 12.1) construction
  line L5 (-52.02, 7.9) -> (-62.22, 12.1) construction
  line L6 (-32.24, 4.9) -> (-22.04, 4.9)
  line L7 (-22.04, 4.9) -> (-22.04, 9.1)
  line L8 (-22.04, 9.1) -> (-32.24, 9.1)
  line L9 (-32.24, 9.1) -> (-32.24, 4.9)
  line L10 (-32.24, 4.9) -> (-22.04, 9.1) construction
  line L11 (-22.04, 4.9) -> (-32.24, 9.1) construction
  line L12 (105.1, -7.9) -> (94.9, -7.9)
  line L13 (94.9, -7.9) -> (94.9, -12.1)
  line L14 (94.9, -12.1) -> (105.1, -12.1)
  line L15 (105.1, -12.1) -> (105.1, -7.9)
  line L16 (105.1, -7.9) -> (94.9, -12.1) construction
  line L17 (94.9, -7.9) -> (105.1, -12.1) construction
  line L18 (55.1, -2.9) -> (44.9, -2.9)
  line L19 (44.9, -2.9) -> (44.9, -7.1)
  line L20 (44.9, -7.1) -> (55.1, -7.1)
  line L21 (55.1, -7.1) -> (55.1, -2.9)
  line L22 (55.1, -2.9) -> (44.9, -7.1) construction
  line L23 (44.9, -2.9) -> (55.1, -7.1) construction
  point P0 (0, 0)
  point P1 (187.2729, -30.3412)
  point P2 (186.9571, -30.2185)
  point P3 (186.5156, -30.047)
  point P4 (185.9486, -29.8268)
  point P5 (185.2566, -29.5592)
  point P6 (184.44, -29.2438)
  point P7 (183.4996, -28.8819)
  point P8 (182.4363, -28.4739)
  point P9 (181.2511, -28.0211)
  point P10 (179.9446, -27.524)
  point P11 (178.5185, -26.9837)
  point P12 (176.9735, -26.4013)
  point P13 (175.3114, -25.7779)
  point P14 (173.5331, -25.115)
  point P15 (171.6406, -24.4138)
  point P16 (169.6356, -23.6757)
  point P17 (167.5195, -22.9016)
  point P18 (165.2943, -22.0936)
  point P19 (162.9622, -21.2532)
  point P20 (160.5252, -20.3816)
  point P21 (157.9852, -19.4805)
  point P22 (155.345, -18.5515)
  point P23 (152.6064, -17.5964)
  point P24 (149.7725, -16.617)
  point P25 (146.8453, -15.6145)
  point P26 (143.8281, -14.591)
  point P27 (140.723, -13.5481)
  point P28 (137.5335, -12.4879)
  point P29 (134.2619, -11.4116)
  point P30 (130.9118, -10.3215)
  point P31 (127.4861, -9.2191)
  point P32 (123.9882, -8.1063)
  point P33 (120.421, -6.9848)
  point P34 (116.7883, -5.8565)
  point P35 (113.093, -4.7232)
  point P36 (109.339, -3.5868)
  point P37 (105.53, -2.4491)
  point P38 (101.6692, -1.3119)
  point P39 (97.7605, -0.177)
  point P40 (93.8074, 0.9538)
  point P41 (89.8141, 2.0788)
  point P42 (85.7842, 3.196)
  point P43 (81.7215, 4.3034)
  point P44 (77.6302, 5.3994)
  point P45 (73.5137, 6.4825)
  point P46 (69.3766, 7.5503)
  point P47 (65.2225, 8.6015)
  point P48 (61.0558, 9.6342)
  point P49 (56.8801, 10.6469)
  point P50 (52.6999, 11.6375)
  point P51 (48.519, 12.6044)
  point P52 (44.3416, 13.5464)
  point P53 (40.1718, 14.4614)
  point P54 (36.0138, 15.348)
  point P55 (31.8716, 16.2046)
  point P56 (27.7292, 17.0318)
  point P57 (23.5957, 17.8204)
  point P58 (19.4889, 18.5665)
  point P59 (15.4127, 19.2689)
  point P60 (11.3715, 19.9265)
  point P61 (7.3697, 20.539)
  point P62 (3.4115, 21.105)
  point P63 (-0.4991, 21.6249)
  point P64 (-4.3576, 22.0972)
  point P65 (-8.1602, 22.5223)
  point P66 (-11.9026, 22.8997)
  point P67 (-15.581, 23.2295)
  point P68 (-19.1913, 23.5114)
  point P69 (-22.7298, 23.746)
  point P70 (-26.1924, 23.9333)
  point P71 (-29.5754, 24.0738)
  point P72 (-32.8755, 24.1679)
  point P73 (-36.0887, 24.2166)
  point P74 (-39.2115, 24.2203)
  point P75 (-42.2412, 24.1801)
  point P76 (-45.1739, 24.0966)
  point P77 (-48.0067, 23.9713)
  point P78 (-50.7365, 23.8049)
  point P79 (-53.3606, 23.5984)
  point P80 (-55.876, 23.3537)
  point P81 (-58.2801, 23.0714)
  point P82 (-60.5704, 22.7531)
  point P83 (-62.7448, 22.4002)
  point P84 (-64.8007, 22.0138)
  point P85 (-66.7361, 21.5955)
  point P86 (-68.5491, 21.1466)
  point P87 (-70.238, 20.6682)
  point P88 (-71.8008, 20.1617)
  point P89 (-73.2366, 19.6284)
  point P90 (-74.5434, 19.0696)
  point P91 (-75.7203, 18.4861)
  point P92 (-76.7666, 17.8795)
  point P93 (-77.6807, 17.25)
  point P94 (-78.4624, 16.5991)
  point P95 (-79.1112, 15.9276)
  point P96 (-79.6262, 15.2359)
  point P97 (-80.0073, 14.5246)
  point P98 (-80.2548, 13.7943)
  point P99 (-80.3681, 13.0456)
  point P100 (-80.3472, 12.2885)
  point P101 (-80.1915, 11.5335)
  point P102 (-79.9018, 10.781)
  point P103 (-79.4785, 10.031)
  point P104 (-78.9223, 9.2838)
  point P105 (-78.2341, 8.5403)
  point P106 (-77.4147, 7.8002)
  point P107 (-76.4655, 7.064)
  point P108 (-75.3874, 6.3322)
  point P109 (-74.1818, 5.6053)
  point P110 (-72.8502, 4.8838)
  point P111 (-71.3939, 4.1679)
  point P112 (-69.8149, 3.4582)
  point P113 (-68.1146, 2.7549)
  point P114 (-66.2953, 2.0587)
  point P115 (-64.3585, 1.3696)
  point P116 (-62.3065, 0.6884)
  point P117 (-60.1415, 0.015)
  point P118 (-57.8656, -0.6503)
  point P119 (-55.4811, -1.3068)
  point P120 (-52.9907, -1.9544)
  point P121 (-50.3966, -2.5935)
  point P122 (-47.7017, -3.2231)
  point P123 (-44.9086, -3.8439)
  point P124 (-42.0197, -4.4556)
  point P125 (-39.0383, -5.0583)
  point P126 (-35.9673, -5.6522)
  point P127 (-32.8096, -6.2371)
  point P128 (-29.568, -6.8139)
  point P129 (-26.2459, -7.382)
  point P130 (-22.8466, -7.9426)
  point P131 (-19.3732, -8.4954)
  point P132 (-15.8289, -9.0413)
  point P133 (-12.2176, -9.5808)
  point P134 (-8.5419, -10.1139)
  point P135 (-4.8063, -10.6416)
  point P136 (-1.0138, -11.1643)
  point P137 (2.832, -11.6824)
  point P138 (6.7273, -12.197)
  point P139 (10.6682, -12.7086)
  point P140 (14.6511, -13.2174)
  point P141 (18.6722, -13.7244)
  point P142 (22.7276, -14.2298)
  point P143 (26.8269, -14.736)
  point P144 (30.9731, -15.2377)
  point P145 (35.1422, -15.7311)
  point P146 (39.3308, -16.2158)
  point P147 (43.5338, -16.6923)
  point P148 (47.7478, -17.1614)
  point P149 (51.9685, -17.6229)
  point P150 (56.1911, -18.0771)
  point P151 (60.4119, -18.5244)
  point P152 (64.6267, -18.9647)
  point P153 (68.8312, -19.3986)
  point P154 (73.0211, -19.8258)
  point P155 (77.1923, -20.2469)
  point P156 (81.3405, -20.6615)
  point P157 (85.4621, -21.0696)
  point P158 (89.5522, -21.4718)
  point P159 (93.607, -21.8674)
  point P160 (97.6228, -22.2564)
  point P161 (101.5953, -22.6392)
  point P162 (105.5203, -23.0151)
  point P163 (109.3943, -23.3844)
  point P164 (113.2132, -23.7466)
  point P165 (116.973, -24.1015)
  point P166 (120.6703, -24.449)
  point P167 (124.3014, -24.789)
  point P168 (127.862, -25.1212)
  point P169 (131.3491, -25.445)
  point P170 (134.7593, -25.7604)
  point P171 (138.0886, -26.0674)
  point P172 (141.334, -26.3652)
  point P173 (144.4922, -26.654)
  point P174 (147.5598, -26.9334)
  point P175 (150.5339, -27.2033)
  point P176 (153.4115, -27.4631)
  point P177 (156.1894, -27.713)
  point P178 (158.8649, -27.9527)
  point P179 (161.4353, -28.1818)
  point P180 (163.8978, -28.4004)
  point P181 (166.25, -28.6084)
  point P182 (168.4895, -28.8053)
  point P183 (170.6138, -28.9915)
  point P184 (172.6208, -29.1666)
  point P185 (174.5085, -29.3303)
  point P186 (176.2747, -29.4831)
  point P187 (177.9179, -29.6247)
  point P188 (179.436, -29.7548)
  point P189 (180.8275, -29.8737)
  point P190 (182.091, -29.9812)
  point P191 (183.2249, -30.0776)
  point P192 (184.2285, -30.1624)
  point P193 (185.1005, -30.236)
  point P194 (185.8397, -30.2983)
  point P195 (186.4459, -30.3491)
  point P196 (186.9179, -30.3889)
  point P197 (187.2554, -30.417)
  point P198 (187.458, -30.434)
  point P199 (-57.12, 10)
  dimension "d14" = 10.3
  dimension "d15" = 81.42
  dimension "d81" = 10.2
  dimension "d82" = 4.2
  dimension "d84" = 10.2
  dimension "d85" = 4.2
  dimension "d87" = 0
  dimension "d151" = 57.12
  dimension "d152" = 10
  dimension "d153" = 27.14
  dimension "d154" = 7
  dimension "d243" = 10.2
  dimension "d244" = 4.2
  dimension "d245" = 100
  dimension "d246" = 10
  dimension "d247" = 10.2
  dimension "d248" = 4.2
  dimension "d249" = 50
  dimension "d250" = 5
  constraints: 48 end point, 8 midpoint, 8 parallel, 4 horizontal, 4 perpendicular, 1 centre point, 201 other
  measures "d14" diameter of A0
  measures "d15" distance of A0.centre point (-80.368, 13.046)
  measures "d81" distance of L2.end L1.end
  measures "d82" distance of L1.end L0.end
  measures "d84" distance of L8.end L7.end
  measures "d85" distance of L7.end L6.end
  measures "d87" distance of point (0, 0) A0.centre
  measures "d151" horizontal distance of point (0, 0) point (-57.12, 10)
  measures "d152" vertical distance of A0.centre point (-57.12, 10)
  measures "d153" horizontal distance of point (0, 0) point (-27.14, 7)
  measures "d154" vertical distance of point (0, 0) point (-27.14, 7)
  measures "d243" distance of L14.end L13.end
  measures "d244" distance of L13.end L12.end
  measures "d245" horizontal distance of point (0, 0) point (100, -10)
  measures "d246" vertical distance of point (0, 0) point (100, -10)
  measures "d247" distance of L20.end L19.end
  measures "d248" distance of L19.end L18.end
  measures "d249" horizontal distance of point (0, 0) point (50, -5)
  measures "d250" vertical distance of point (0, 0) point (50, -5)